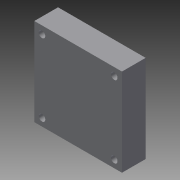
# Autodesk Inventor part: ventilator
Saved by Autodesk Inventor 2013 (Build 170138000, 138)
## iProperties
Created: 2015-06-08
Part Number: ventilator
Material: Generic
Document SubType Name: Modeling
Designer: Jufo
Density: 1 g/cm^3
Author: Jufo
Autodesk Inventor part; units mm, degrees
ref_plane "YZ Plane" through (0, 0, 0) normal (1, 0, 0) x (0, 1, 0)
ref_plane "XZ Plane" through (0, 0, 0) normal (0, 1, 0) x (-1, 0, 0)
ref_plane "XY Plane" through (0, 0, 0) normal (0, 0, 1) x (1, 0, 0)
sketch "Sketch1" plane through (0, 0, 0) normal (0, 1, 0) x (-1, 0, 0)
  line L0 (-22.0009, 16.7182) -> (-22.0009, -23.1818)
  line L1 (-22.0009, -23.1818) -> (17.8991, -23.1818)
  line L2 (17.8991, -23.1818) -> (17.8991, 16.7182)
  line L3 (17.8991, 16.7182) -> (-22.0009, 16.7182)
  circle A0 centre (14.3991, -19.6818) radius 1.5
  circle A1 centre (14.4378, 13.2182) radius 1.5
  circle A2 centre (-18.5009, 13.2182) radius 1.5
  circle A3 centre (-18.5009, -19.6818) radius 1.5
  point P0 (0, 0)
  dimension "d0" = 39.9
  dimension "d2" = 39.9
  dimension "d3" = 3
  dimension "d4" = 3
  dimension "d5" = 3
  dimension "d6" = 3
  dimension "d7" = 3.5
  dimension "d8" = 3.5
  dimension "d9" = 3.5
  dimension "d10" = 3.5
  dimension "d11" = 3.5
  dimension "d12" = 3.5
  dimension "d13" = 3.5
  constraints: 8 end point, 4 centre point, 2 parallel, 1 perpendicular, 1 vertical
  measures "d0" distance of L2.end L0.start
  measures "d2" distance of L1.end L2.end
  measures "d3" diameter of A0
  measures "d4" diameter of A3
  measures "d5" diameter of A2
  measures "d6" diameter of A1
  measures "d7" distance from line of L3 A2.centre
  measures "d8" distance from line of L1 A3.centre
  measures "d9" distance from line of L1 A0.centre
  measures "d10" distance from line of L3 A1.centre
  measures "d11" distance from line of L0 A2.centre
  measures "d12" distance from line of L0 A3.centre
  measures "d13" distance from line of L2 A0.centre
extrude "Extrusion1" add sketch "Sketch1" along normal blind 10.8
body "Solid1"
